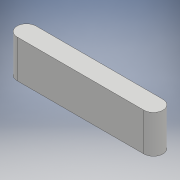
# Autodesk Inventor part: Key
Saved by Autodesk Inventor 2018 (Build 220112000, 112)
## iProperties
Created: 2017-06-01
Part Number: Key
Material: Generic
Document SubType Name: Modeling
Designer: Mikołaj
Density: 1 g/cm^3
Appearance: Default
Mass: 0.032857 g
Surface Area: 0.811332 cm^2
Volume: 0.032857 cm^3
Author: Mikołaj
Autodesk Inventor part; units mm, degrees
ref_plane "YZ Plane" through (0, 0, 0) normal (1, 0, 0) x (0, 1, 0)
ref_plane "XZ Plane" through (0, 0, 0) normal (0, 1, 0) x (-1, 0, 0)
ref_plane "XY Plane" through (0, 0, 0) normal (0, 0, 1) x (1, 0, 0)
sketch "Sketch1" plane through (0, 0, 0) normal (0, 0, 1) x (1, 0, 0)
  line L0 (-4.35, 0.65) -> (4.35, 0.65)
  line L1 (-4.35, -0.65) -> (4.35, -0.65)
  arc A0 (4.35, -0.65) -> (4.35, 0.65) centre (4.35, 0) ccw
  arc A1 (-4.35, 0.65) -> (-4.35, -0.65) centre (-4.35, 0) ccw
  dimension "d0" = 1.3
  dimension "d1" = 10
  dimension "d2" = 8.7
  constraints: 4 end point, 4 point on circle, 2 centre point, 2 horizontal, 2 tangent
  measures "d0" distance between parallel lines of L1 L0
  measures "d2" distance of A0.centre A1.centre
extrude "Extrusion1" add sketch "Sketch1" along normal blind 2.6
body "Solid1"
